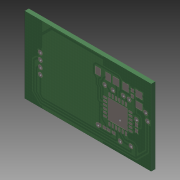
# Autodesk Inventor part: NFC_module_PCB
Saved by Autodesk Inventor 2013 (Build 170138000, 138)
## iProperties
Created: 2015-07-04
Part Number: NFC_module_PCB
Material: Ogólny
Document SubType Name: Modeling
Designer: terg
Density: 1 g/cm^3
Author: terg
Autodesk Inventor part; units mm, degrees
ref_plane "YZ Plane" through (0, 0, 0) normal (1, 0, 0) x (0, 1, 0)
ref_plane "XZ Plane" through (0, 0, 0) normal (0, 1, 0) x (-1, 0, 0)
ref_plane "XY Plane" through (0, 0, 0) normal (0, 0, 1) x (1, 0, 0)
sketch "Szkic1" plane through (0, 0, 0) normal (0, 1, 0) x (-1, 0, 0)
  line L0 (0, 0) -> (25, 0)
  line L1 (25, 0) -> (25, 15)
  line L2 (25, 15) -> (0, 15)
  line L3 (0, 15) -> (0, 0)
  dimension "d0" = 25
  dimension "d1" = 15
  constraints: 8 end point, 2 parallel, 1 horizontal, 1 perpendicular
  measures "d0" distance of L2.end L1.end
  measures "d1" distance of L1.end L0.end
extrude "Wyciągnięcie proste1" add sketch "Szkic1" along normal blind 0.8
sketch "Szkic2" plane through (0, 0.8, 0) normal (0, 1, 0) x (1, 0, 0)
  line L0 (0, 0) -> (-25, 0) projected
  line L1 (-25, 0) -> (-25, -15) projected
  line L2 (-25, -15) -> (0, -15) projected
  line L3 (0, -15) -> (0, 0) projected
  line L4 (-25.0063, 0) -> (0.0063, 0) construction
  line L5 (0.0063, 0) -> (0.0063, -15) construction
  line L6 (0.0063, -15) -> (-25.0063, -15) construction
  line L7 (-25.0063, -15) -> (-25.0063, 0) construction
  dimension "d9" = 0
  dimension "d10" = -0.0063
  dimension "d11" = 0
  dimension "d12" = -0.0063
  constraints: 2 other
  measures "d9" distance between parallel lines of L0 L4
  measures "d10" distance between parallel lines of L3 L5
  measures "d11" distance between parallel lines of L2 L6
  measures "d12" distance between parallel lines of L1 L7
decal "Pokrycie bitmapą1"
sketch "Szkic3" plane through (0, 0, 0) normal (0, -1, 0) x (1, 0, 0)
  line L0 (0, 0) -> (-25, 0) projected
  line L1 (0, 15) -> (0, 0) projected
  line L2 (-25, 15) -> (0, 15) projected
  line L3 (-25, 0) -> (-25, 15) projected
  line L4 (-0.0125, 0) -> (-24.9875, 0) construction
  line L5 (-24.9875, 0) -> (-24.9875, 15) construction
  line L6 (-24.9875, 15) -> (-0.0125, 15) construction
  line L7 (-0.0125, 15) -> (-0.0125, 0) construction
  dimension "d25" = 0
  dimension "d26" = 0.0125
  dimension "d28" = 0
  dimension "d29" = 0.0125
  constraints: 2 other
  measures "d25" distance between parallel lines of L0 L4
  measures "d26" distance between parallel lines of L1 L7
  measures "d28" distance between parallel lines of L2 L6
  measures "d29" distance between parallel lines of L3 L5
decal "Pokrycie bitmapą2"
sketch "Szkic4" plane through (0, 0.8, 0) normal (0, 1, 0) x (1, 0, 0)
  point P0 (-21.9046, -5.6225)
  point P1 (-21.9046, -6.8544)
  point P2 (-21.9046, -8.1299)
  point P3 (-21.9046, -9.4199)
  point P4 (-10.5234, -2.6855)
  point P5 (-6.137, -2.0933)
  point P6 (-4.0095, -2.2907)
  point P7 (-6.1975, -5.6966)
  point P8 (-2.889, -7.4066)
  point P9 (-0.6797, -8.2272)
  point P10 (-9.1745, -10.2298)
  point P11 (-7.5525, -10.1225)
  point P12 (-5.4957, -10.1997)
  point P13 (-4.3484, -10.1305)
  point P14 (-1.0886, -9.5034)
hole "Otwór1" at (-21.9046, 0.8, 5.6225) at (-21.9046, 0.8, 6.8544) at (-21.9046, 0.8, 8.1299) at (-21.9046, 0.8, 9.4199) at (-10.5234, 0.8, 2.6855) at (-6.137, 0.8, 2.0933) at (-4.0095, 0.8, 2.2907) at (-6.1975, 0.8, 5.6966) at (-2.889, 0.8, 7.4066) at (-0.6797, 0.8, 8.2272) at (-9.1745, 0.8, 10.2298) at (-7.5525, 0.8, 10.1225) at (-5.4957, 0.8, 10.1997) at (-4.3484, 0.8, 10.1305) at (-1.0886, 0.8, 9.5034) direction (0, -1, 0) diameter 0.4 depth 8
equation "\"d10\" = d12"
equation "\"d26\" = d29"
